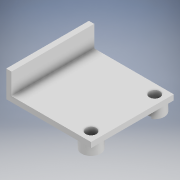
# Autodesk Inventor part: DržačSenzoraUdaljenostiOnlyOne(1)_v.1.0
Saved by Autodesk Inventor 2020 (Build 240168000, 168)
## iProperties
Created: 2020-07-11
Part Number: DržačSenzoraUdaljenostiOnlyOne(1)_v.1.0
Material: Generic
Document SubType Name: Modeling
Designer: Sičaja
Density: 1 g/cm^3
Appearance: Default
Author: Sičaja
Autodesk Inventor part; units mm, degrees
ref_plane "YZ Plane" through (0, 0, 0) normal (1, 0, 0) x (0, 1, 0)
ref_plane "XZ Plane" through (0, 0, 0) normal (0, 1, 0) x (-1, 0, 0)
ref_plane "XY Plane" through (0, 0, 0) normal (0, 0, 1) x (1, 0, 0)
sketch "Sketch1" plane through (0, 0, 0) normal (0, 1, 0) x (-1, 0, 0)
  circle A0 centre (0, 6) radius 1
  circle A1 centre (0, -6) radius 1
  line L0 (0, -7.8) -> (-1.8, -7.8)
  line L1 (0, 7.8) -> (-1.8, 7.8)
  line L2 (-1.8, 7.8) -> (-1.8, -7.8)
  line L3 (-1.8, 7.8) -> (12.2, 7.8)
  line L4 (12.2, 7.8) -> (12.2, -7.8)
  line L5 (12.2, -7.8) -> (-1.8, -7.8)
  line L6 (0, 6) -> (1.8, 6)
  line L7 (1.8, 7.8) -> (1.8, -7.8)
  arc A2 (1.2036, -6.4912) -> (-0.6275, -4.8615) centre (0, -6) ccw
  circle A3 centre (0, 6) radius 1.8
  arc A4 (-0.9, -4.4412) -> (1.6551, -6.7077) centre (0, -6) ccw
  line L8 (-0.9, -4.4412) -> (-0.6275, -4.8615)
  line L9 (1.2036, -6.4912) -> (1.6551, -6.7077)
  line L10 (12.2, -7.8) -> (13.2, -7.8)
  line L11 (13.2, -7.8) -> (13.2, 7.8)
  line L12 (13.2, 7.8) -> (12.2, 7.8)
  line L13 (12.2, 7.8) -> (12.2, -7.8)
  line L14 (13.2, -7.8) -> (14.2, -7.8)
  line L15 (14.2, -7.8) -> (14.2, 7.8)
  line L16 (14.2, 7.8) -> (13.2, 7.8)
  line L17 (13.2, -7.8) -> (14.2, -7.8)
  point P0 (0, 0)
  dimension "d2" = 2
  dimension "d3" = 2
  dimension "d4" = 1.8
  dimension "d5" = 1.8
  dimension "d6" = 1.8
  dimension "d7" = 1.8
  dimension "d8" = 14
  dimension "d9" = 1.8
  dimension "d10" = 2.6
  dimension "d11" = 3.6
  dimension "d12" = 3.6
  dimension "d13" = 1
  dimension "d14" = 1
  constraints: 36 end point, 6 perpendicular, 5 centre point, 5 horizontal, 4 point on circle, 3 coincident, 2 collinear, 2 point on line, 1 vertical
  measures "d2" diameter of A0
  measures "d3" diameter of A1
  measures "d4" distance of A1.centre L0.start
  measures "d5" distance of L0.start L0.end
  measures "d6" distance of L6.start L1.start
  measures "d7" distance of L1.start L1.end
  measures "d8" distance of L1.end L3.end
  measures "d9" distance of L6.start L6.end
  measures "d10" diameter of A2
  measures "d11" diameter of A3
  measures "d12" diameter of A4
  measures "d13" distance of L4.end L10.end
  measures "d14" distance of L10.end L14.end
extrude "Extrusion1" add sketch "Sketch1" along normal blind 1.8 contours A4 L8 A2 L9 | A3
sketch "Sketch2" plane through (0, 1.8, 6) normal (0, 1, 0) x (1, 0, 0)
  circle A0 centre (0, 0) radius 1 projected
  line L0 (0, 0) -> (1.8, 0)
  circle A1 centre (0, 0) radius 1.8 projected
  line L1 (1.8, 0) -> (1.8, -1.8)
  arc A2 (0.9, 10.4412) -> (-1.6551, 12.7077) centre (0, 12) ccw projected
  line L2 (1.8, 13.8) -> (0, 13.8)
  line L3 (1.8, 13.8) -> (1.8, -1.8)
  line L4 (0, 0) -> (-1.8, 0)
  line L5 (-1.8, 0) -> (-1.8, -1.8)
  line L6 (-1.8, -1.8) -> (1.8, -1.8)
  line L7 (-1.8, -1.8) -> (-1.8, 12.0403)
  line L8 (-1.8, 12.0403) -> (-1.8, 13.8)
  line L9 (-1.8, 13.8) -> (0, 13.8)
  line L10 (-1.8, 13.8) -> (-1.8, -1.8)
  line L11 (-1.8, -1.8) -> (1.8, -1.8)
  arc A3 (-1.2036, 12.4912) -> (0.6275, 10.8615) centre (0, 12) ccw projected
  line L12 (0.6275, 10.8615) -> (0.9, 10.4412) projected
  arc A4 (0.9, 10.4412) -> (-1.6551, 12.7077) centre (0, 12) ccw projected
  line L13 (-1.6551, 12.7077) -> (-1.2036, 12.4912) projected
  arc A5 (-1.2036, 12.4912) -> (0.6275, 10.8615) centre (0, 12) ccw projected
  circle A6 centre (0, 12) radius 1 projected
  point P0 (0, 6)
  dimension "d18" = 1.8
  constraints: 24 end point, 3 collinear, 3 tangent, 2 horizontal, 2 perpendicular, 2 point on circle, 2 vertical, 1 point on line
  measures "d18" distance of L0.start L0.end
extrude "Extrusion2" add sketch "Sketch2" along normal blind 1 contours L0 A1 L4 A0 | A0 L4 A1 L0 | L1 L6 A1 | A1 L7 L8 L9 A2 L13 A3 L12 L3 | A1 L6 L5 | A2 L12 A3 L13 | A2 L2 L3
sketch "Sketch3" plane through (-1.8, 1.8, -7.8) normal (-1, 0, 0) x (0, 0, 1)
  line L0 (0, 0) -> (13.8, 0) projected
  line L1 (13.8, 0) -> (15.6, 0) projected
  line L2 (15.6, 0) -> (15.6, 1) projected
  line L3 (0, 1) -> (15.6, 1) projected
  line L4 (0, 0) -> (0, 1) projected
  point P0 (7.8, -1.8)
extrude "Extrusion3" add sketch "Sketch3" along normal blind 12.4
sketch "Sketch4" plane through (0, 2.8, 6) normal (0, 1, 0) x (1, 0, 0)
  line L0 (-14.2, 13.8) -> (-14.2, -1.8) projected
  line L1 (-14.2, -1.8) -> (-14.2, 13.8)
  line L2 (-14.2, 13.8) -> (-13.2, 13.8)
  line L3 (1.8, 13.8) -> (-14.2, 13.8) projected
  line L4 (-13.2, 13.8) -> (-13.2, -1.8)
  line L5 (1.8, -1.8) -> (-14.2, -1.8) projected
  point P0 (0, 6)
  dimension "d23" = 1
  constraints: 6 end point, 2 point on line, 1 collinear, 1 perpendicular
  measures "d23" distance of L0.start L2.end
extrude "Extrusion4" add sketch "Sketch4" along normal blind 4
body "Solid1"
